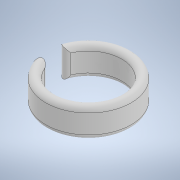
# Autodesk Inventor part: CableRing
Saved by Autodesk Inventor 2020 (Build 240168000, 168)
## iProperties
Created: 2020-07-04
Part Number: CableRing
Material: Generic
Document SubType Name: Modeling
Designer: maple
Density: 1 g/cm^3
Appearance: Default
Author: maple
Autodesk Inventor part; units mm, degrees
ref_plane "YZ Plane" through (0, 0, 0) normal (1, 0, 0) x (0, 1, 0)
ref_plane "XZ Plane" through (0, 0, 0) normal (0, 1, 0) x (-1, 0, 0)
ref_plane "XY Plane" through (0, 0, 0) normal (0, 0, 1) x (1, 0, 0)
sketch "Sketch1" plane through (0, 0, 0) normal (0, 1, 0) x (-1, 0, 0)
  circle A0 centre (0, 0) radius 7
  circle A1 centre (0, 0) radius 9
  line L0 (7, 0) -> (9, 0)
  line L1 (9, 0) -> (8.6528, -2.4758)
  line L2 (9, 0) -> (8.6528, 2.4758)
  line L3 (8.6528, 2.4758) -> (0, 0)
  line L4 (0, 0) -> (8.6528, -2.4758)
  point P0 (6.7299, -1.9256)
  point P1 (6.7299, 1.9256)
  dimension "d0" = 14
  dimension "d1" = 18
  dimension "d2" = 2.5
  dimension "d3" = 2.5
  constraints: 10 end point, 3 point on circle, 2 coincident, 1 centre point, 1 horizontal, 3 other
  measures "d1" diameter of A1
  measures "d2" distance of L0.end L1.end
  measures "d3" distance of L0.end L2.end
extrude "Extrusion1" add sketch "Sketch1" along normal blind 6 contours A0 L4 A1 L3
fillet "Fillet1" radius 1 8 edges at (7, 0, 0) (9, 0, 0) (9, 6, 0) (7, 6, 0) (-8.6528, 3, -2.4758) (-6.7299, 3, -1.9256) (-8.6528, 3, 2.4758) (-6.7299, 3, 1.9256)
body "Solid1"
